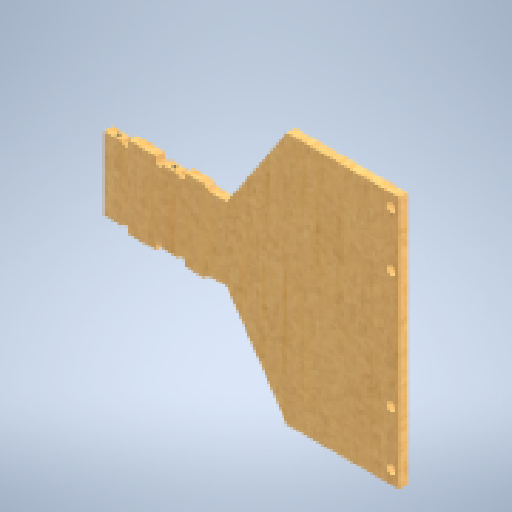
# Autodesk Inventor part: hera_porika2
Saved by Autodesk Inventor 2024 (Build 280153000, 153)
## iProperties
Created: 2024-01-03
Part Number: hera_porika2
Material: ポリカーボネート、クリア
Document SubType Name: Modeling
Designer: right
Density: 1.2 g/cm^3
Appearance: イエロー パイン材 - 硬質 塗装 抑えた光沢
Mass: 11.4076 g
Surface Area: 146.016 cm^2
Volume: 9.50636 cm^3
Author: right
Autodesk Inventor part; units mm, degrees
ref_plane "YZ Plane" through (0, 0, 0) normal (1, 0, 0) x (0, 1, 0)
ref_plane "XZ Plane" through (0, 0, 0) normal (0, 1, 0) x (-1, 0, 0)
ref_plane "XY Plane" through (0, 0, 0) normal (0, 0, 1) x (1, 0, 0)
sketch "スケッチ1" plane through (0, 0, 0) normal (0, 0, 1) x (1, 0, 0)
  line L0 (-10.8, 27.5) -> (31.8, 27.5)
  line L1 (31.8, 27.5) -> (31.8, 1.5)
  line L2 (31.8, 1.5) -> (-10.8, 1.5)
  line L3 (-10.8, 1.5) -> (-10.8, 27.5)
  line L4 (-35.2, 27.5) -> (27.8, 27.5) projected
  line L5 (-35.2, 1.5) -> (27.8, 1.5) projected
  line L6 (-8.3, 29) -> (-6.1, 29) projected
  line L7 (31.8, 1.5) -> (27.8, 1.5) projected
  ellipse E0 centre (-172.2553, 12.25) end of major axis (-172.2553, 4.25) minor radius 7.9976 projected
  line L8 (94.2, 59.5) -> (94.2, -30.5)
  line L9 (31.8, 14.5) -> (94.2, 14.5) construction
  line L10 (94.2, 59.5) -> (54.2, 59.5)
  line L11 (31.8, 27.5) -> (32.8, 27.5)
  line L12 (32.8, 27.5) -> (54.2, 59.5)
  circle A0 centre (32.2657, 28.5) radius 1
  line L13 (94.2, -30.5) -> (54.2, -30.5)
  line L14 (31.8, 2.9953) -> (54.2, -30.5)
  line L15 (0, 0) -> (5.6, 0) projected
  line L16 (5.6, 0) -> (5.6, 1.5) projected
  line L17 (0, 1.5) -> (5.6, 1.5) projected
  line L18 (0, 0) -> (0, 1.5) projected
  line L19 (-2.2, 1.5) -> (0, 1.5) projected
  line L20 (-2.2, 0) -> (0, 0) projected
  line L21 (5.6, 0) -> (7.8, 0) projected
  line L22 (11.7, 0) -> (13.9, 0) projected
  line L23 (17.8, 0) -> (20, 0) projected
  line L24 (20, 0) -> (25.6, 0) projected
  line L25 (25.6, 0) -> (27.8, 0) projected
  line L26 (17.8, 0) -> (17.8, 1.5)
  line L27 (31.8, 1.5) -> (32.8, 1.5)
  line L28 (27.8, 0) -> (27.8, 1.5)
  arc A1 (24.6775, 0) -> (27.8, 1.5) centre (24.6775, 4) ccw
  arc A2 (27.8, 1.5) -> (24.6775, 0) centre (27.8, -2.5) ccw
  circle A3 centre (16.7, 1.5) radius 1.1
  line L29 (7.8, 0) -> (7.8, 1.5)
  line L30 (-2.2, 0) -> (-2.2, 1.5)
  circle A4 centre (8.9, 1.5) radius 1.1
  circle A5 centre (-3.3, 1.5) radius 1.1
  line L31 (0, 29) -> (5.6, 29)
  line L32 (5.6, 29) -> (5.6, 27.5)
  line L33 (0, 29) -> (0, 27.5)
  line L34 (-2.2, 29) -> (0, 29)
  line L35 (11.7, 29) -> (13.9, 29)
  line L36 (17.8, 29) -> (20, 29)
  line L37 (20, 29) -> (25.6, 29)
  line L38 (25.6, 29) -> (27.8, 29)
  line L39 (17.8, 29) -> (17.8, 27.5)
  line L40 (27.8, 29) -> (27.8, 27.5)
  arc A6 (27.8, 27.5) -> (24.6775, 29) centre (24.6775, 25) ccw
  arc A7 (24.6775, 29) -> (27.8, 27.5) centre (27.8, 31.5) ccw
  circle A8 centre (16.7, 27.5) radius 1.1
  line L41 (-2.2, 29) -> (-2.2, 27.5)
  circle A9 centre (8.9, 27.5) radius 1.1
  line L42 (0, 29) -> (5.6, 29)
  line L43 (5.6, 29) -> (5.6, 27.5)
  line L44 (0, 29) -> (0, 27.5)
  line L45 (-2.2, 29) -> (0, 29)
  line L46 (5.6, 29) -> (7.8, 29)
  line L47 (7.8, 29) -> (7.8, 27.5)
  line L48 (-2.2, 29) -> (-2.2, 27.5)
  circle A10 centre (-3.3, 27.5) radius 1.1
  point P0 (15.6, 27.5)
  point P1 (10, 27.5)
  point P2 (7.8, 27.5)
  point P3 (-4.4, 1.5)
  point P4 (10, 1.5)
  point P5 (15.6, 1.5)
  point P6 (7.8, 27.5)
  point P7 (-4.4, 27.5)
  dimension "d7" = 2.2
  dimension "d8" = 2.2
  dimension "d9" = 2.2
  dimension "d0" = 2.5
  dimension "d2" = 1
  dimension "d3" = 2
  dimension "d4" = 90
  dimension "d5" = 40
  dimension "d6" = 4
  dimension "d39" = 105
  constraints: 68 end point, 24 symmetric about line, 12 point on line, 8 point on circle, 7 centre point, 5 horizontal, 4 perpendicular, 4 tangent, 3 parallel, 2 midpoint, 2 vertical, 17 other
  measures "d0" distance from line of L3 L6.start
  measures "d2" distance of L0.end L11.end
  measures "d3" diameter of A0
  measures "d4" distance of L8.start L8.end
  measures "d5" distance of L8.start L10.end
  measures "d6" radius of A1
  measures "d39" distance between parallel lines of L8 L3
extrude "押し出し1" add sketch "スケッチ1" along normal blind 3 contours L41 L34 L33 L0 | L0 A9 A8 L1 L2 A3 A4 A5 L3 A10 | L33 L31 L32 L0 | L32 L46 L47 L0 | L2 L18 L20 L30 | L39 L36 L37 A7 L0 | L2 L16 L15 L18 | L2 L29 L21 L16 | L11 L12 L10 L8 L13 L14 L1 | L14 L27 L1 | A2 L24 L23 L26 L2
fillet "フィレット1" radius 2 2 edges at (32.8, 27.5, 1.5) (32.8, 1.5, 1.5)
sketch "スケッチ2" plane through (0, 0, 0) normal (0, 0, -1) x (-1, 0, 0)
  arc A0 (-33.394, 28.3882) -> (-31.7315, 27.5) centre (-31.7315, 29.5) ccw projected
  arc A1 (-31.7315, 1.5) -> (-33.394, 0.6118) centre (-31.7315, -0.5) ccw projected
  line L0 (-33.394, 28.3882) -> (-33.394, 0.6118)
  line L1 (-54.2, 59.5) -> (-33.394, 28.3882) projected
  line L2 (-94.2, 59.5) -> (-54.2, 59.5) projected
  line L3 (-94.2, -30.5) -> (-94.2, 59.5) projected
  line L4 (-54.2, -30.5) -> (-94.2, -30.5) projected
  line L5 (-33.394, 0.6118) -> (-54.2, -30.5) projected
  arc A2 (-35.8877, 26.7205) -> (-34.1212, 25.1081) centre (-31.7315, 29.5) ccw
  line L6 (-35.8877, 26.7205) -> (-55.8028, 56.5)
  line L7 (-55.8028, 56.5) -> (-91.2, 56.5)
  line L8 (-91.2, 56.5) -> (-91.2, -27.5)
  line L9 (-91.2, -27.5) -> (-55.8028, -27.5)
  line L10 (-55.8028, -27.5) -> (-35.8877, 2.2795)
  arc A3 (-31.7315, 4.5) -> (-35.8877, 2.2795) centre (-31.7315, -0.5) ccw
  line L11 (-38.394, 30.4682) -> (-38.394, -1.4682)
  line L12 (-33.394, 24.4) -> (8.8, 24.4)
  line L13 (8.8, 24.4) -> (8.8, 4.6)
  line L14 (8.8, 4.6) -> (-33.394, 4.6)
  line L15 (-33.394, 4.6) -> (-33.394, 24.4)
  line L16 (10.8, 27.5) -> (10.8, 1.5) projected
  line L17 (-91.2, 14.5) -> (-38.394, 14.5) construction
  line L18 (-33.394, 24.4) -> (8.8, 4.6) construction
  line L19 (8.8, 24.4) -> (-33.394, 4.6) construction
  line L20 (-91.2, 14.5) -> (-45.8453, 41.6103) construction
  line L21 (-91.2, 14.5) -> (-45.8453, -12.6103) construction
  line L22 (-93.0741, 11.6323) -> (-42.432, 41.903)
  line L23 (-42.432, 41.903) -> (-43.9712, 44.478)
  line L24 (-43.9712, 44.478) -> (-94.6133, 14.2073)
  line L25 (-94.6133, 14.2073) -> (-93.0741, 11.6323)
  line L26 (-93.0741, 11.6323) -> (-43.9712, 44.478) construction
  line L27 (-42.432, 41.903) -> (-94.6133, 14.2073) construction
  line L28 (-90.9974, 16.1264) -> (-45.0103, -11.3618)
  line L29 (-46.6802, -13.8587) -> (-94.6133, 14.7927)
  line L30 (-33.395, 3.495) -> (9.6535, 23.696)
  line L31 (9.6535, 23.696) -> (8.8039, 25.5065)
  line L32 (8.8039, 25.5065) -> (-34.2446, 5.3055)
  line L33 (-34.2446, 5.3055) -> (-33.395, 3.495)
  line L34 (-33.395, 3.495) -> (8.8039, 25.5065) construction
  line L35 (9.6535, 23.696) -> (-34.2446, 5.3055) construction
  arc A4 (-15.6, 1.5) -> (-17.8, 1.5) centre (-16.7, 1.5) ccw projected
  arc A5 (-17.8, 27.5) -> (-15.6, 27.5) centre (-16.7, 27.5) ccw projected
  line L36 (8.3403, 3.7125) -> (-33.781, 23.4784)
  line L37 (-33.781, 23.4784) -> (-32.9314, 25.289)
  line L38 (-32.9314, 25.289) -> (9.1899, 5.5231)
  line L39 (9.1899, 5.5231) -> (8.3403, 3.7125)
  line L40 (8.3403, 3.7125) -> (-32.9314, 25.289) construction
  line L41 (-33.781, 23.4784) -> (9.1899, 5.5231) construction
  circle A6 centre (-91.2, 35.5) radius 3
  circle A7 centre (-91.2, 35.5) radius 1.6
  line L42 (-91.2, 56.5) -> (-91.2, 14.5) construction
  circle A8 centre (-91.2, 54.9) radius 3
  circle A9 centre (-91.2, 54.9) radius 1.6
  circle A10 centre (-91.2, -6.5) radius 3
  circle A11 centre (-91.2, -6.5) radius 1.6
  circle A12 centre (-91.2, -25.9) radius 3
  circle A13 centre (-91.2, -25.9) radius 1.6
  circle A14 centre (-73.2, -25.9) radius 1.6
  circle A15 centre (-73.2, -25.9) radius 3
  circle A16 centre (-73.2, 54.9) radius 3
  circle A17 centre (-73.2, 54.9) radius 1.6
  circle A18 centre (-55.2, -25.9) radius 1.6
  circle A19 centre (-55.2, -25.9) radius 3
  circle A20 centre (-55.2, 54.9) radius 3
  circle A21 centre (-55.2, 54.9) radius 1.6
  point P0 (0, 0)
  point P1 (-68.5226, 28.0551)
  point P2 (-93.0741, 17.3677)
  point P3 (-42.432, -12.903)
  point P4 (-43.9712, -15.478)
  point P5 (-12.297, 14.5)
  point P6 (-12.2956, 14.5007)
  point P7 (6.4459, 24.4)
  point P8 (8.8, 23.2954)
  point P9 (-31.0402, 4.6)
  point P10 (-33.394, 5.7047)
  point P11 (-42.7408, -13.697)
  point P12 (-91.2, 12.7525)
  point P13 (-88.2764, 14.5)
  point P14 (-41.3721, -10.9953)
  point P15 (-35.394, 1.2189)
  point P16 (-35.394, 27.7811)
  point P17 (-45.0103, 40.3618)
  point P18 (-91.2, 16.2475)
  point P19 (-46.6802, 42.8587)
  point P20 (-16.7, 2.6)
  point P21 (-16.7, 26.4)
  point P22 (-33.394, 5.7047)
  point P23 (-33.394, 3.4954)
  point P24 (6.4491, 4.6)
  point P25 (-12.2956, 13.3961)
  point P26 (-14.6495, 14.5007)
  point P27 (-33.394, 23.2968)
  point P28 (-9.9416, 14.5007)
  point P29 (8.8, 5.706)
  point P30 (-31.037, 24.4)
  point P31 (-12.2956, 15.6054)
  point P32 (-90.2, 15.4462)
  point P33 (-91.2, 12.7525)
  point P34 (-91.2, 35.5)
  point P35 (-91.2, -6.5)
  point P36 (-91.2, 33.9)
  point P37 (-91.2, 37.1)
  point P38 (-88.6623, 56.5)
  point P39 (-91.2, 51.9)
  point P40 (-91.2, 38.5)
  point P41 (-91.2, 32.5)
  point P42 (-91.2, 53.3)
  point P43 (-91.2, -9.5)
  point P44 (-91.2, -22.9)
  point P45 (-88.6623, -27.5)
  point P46 (-91.2, -3.5)
  point P47 (-91.2, -8.1)
  point P48 (-91.2, -4.9)
  point P49 (-57.7377, -27.5)
  point P50 (-53.2235, -23.6431)
  point P51 (-75.7377, -27.5)
  point P52 (-70.6623, -27.5)
  point P53 (-53.2235, 52.6431)
  point P54 (-57.7377, 56.5)
  point P55 (-70.6623, 56.5)
  point P56 (-75.7377, 56.5)
  point P57 (-55.74, 56.4061)
  point P58 (-54.0143, 53.8257)
  point P59 (-73.2, 56.5)
  point P60 (-55.74, -27.4061)
  point P61 (-54.0143, -24.8257)
  point P62 (-73.2, -27.5)
  dimension "d13" = 3
  dimension "d14" = 5
  dimension "d15" = 2
  dimension "d16" = 3
  dimension "d18" = 2
  dimension "d36" = 2
  dimension "d37" = 2
  dimension "d38" = 2
  dimension "d40" = 6
  dimension "d41" = 3.2
  dimension "d42" = 6
  dimension "d43" = 3.2
  dimension "d48" = 18
  constraints: 74 end point, 18 centre point, 13 midpoint, 12 parallel, 10 point on line, 9 coincident, 9 symmetric about line, 6 point on circle, 4 perpendicular, 3 horizontal, 3 tangent, 1 collinear, 1 vertical, 26 other
  measures "d13" distance between parallel lines of L1 L6
  measures "d14" distance between parallel lines of L0 L11
  measures "d15" distance between parallel lines of L16 L13
  measures "d16" distance of L23.end L22.end
  measures "d18" distance of L31.end L30.end
  measures "d36" distance from line of point (-16.7, 2.6) L14
  measures "d37" distance from line of L12 point (-16.7, 26.4)
  measures "d38" distance of L36.end L37.end
  measures "d40" diameter of A6
  measures "d41" diameter of A7
  measures "d42" diameter of A8
  measures "d43" diameter of A9
  measures "d48" distance of A13.centre A14.centre
extrude "押し出し2" cut sketch "スケッチ2" against normal blind 2 contours L6 L11 L10 L28 L22 | L36 L32 L0 | L12 L32 L38 | L24 L8 A6 A8 L7 A16 A20 L6 | A20 L7 L6 A21 | L29 L10 A19 L9 A15 A12 L8 A10 | L36 L14 L30 | L30 L13 L38 | A21 L6 | A17 | A16 L7 | L8 A7 | A11 L8 | L10 A18 L9 A19 | A9 L8 | L10 A18 | A14 | L9 A15 picked at (-57.4616, 56.0082) picked at (-55.2681, 54.3725) picked at (-70.697, 54.6556) picked at (-90.9686, 35.9805) picked at (-90.783, -6.1675) picked at (-57.4616, -27.0082) picked at (-90.7488, 55.3036) picked at (-55.4528, -26.2997) picked at (-70.697, -25.6556)
fillet "フィレット2" radius 2 29 edges at (91.2, 12.7525, 1) (88.2764, 14.5, 1) (91.2, 16.2475, 1) (46.6802, 42.8587, 1) (45.0103, 40.3618, 1) (33.394, 5.7047, 1) (31.0402, 4.6, 1) (-8.8, 23.2954, 1) (-6.4459, 24.4, 1) (33.394, 23.2968, 1) (31.037, 24.4, 1) (14.6495, 14.5007, 1) (12.2956, 15.6054, 1) (9.9416, 14.5007, 1) (12.2956, 13.3961, 1) (45.0103, -11.3618, 1) (46.6802, -13.8587, 1) (38.394, -1.4682, 1) (38.394, 30.4682, 1) (91.2, -3.5, 1) (91.2, -9.5, 1) (91.2, -22.9, 1) (88.6623, -27.5, 1) (91.2, 38.5, 1) (91.2, 32.5, 1) (91.2, 51.9, 1) (88.6623, 56.5, 1) (55.8028, -27.5, 1) (55.8028, 56.5, 1)
sketch "スケッチ3" plane through (10, 27.5, 0) normal (0, 1, 0) x (1, 0, 0)
  circle A0 centre (2.8, -1.5) radius 1.1 projected
  circle A1 centre (-17.2, -1.5) radius 1.1 projected
  point P0 (-10, 0)
  constraints: 2 coincident
hole "穴1" at (12.8, 27.5, 1.5) at (-7.2, 27.5, 1.5) direction (0, -1, 0) diameter 1.567 depth 4.5 tip angle 118 thread size "M2x0.4" class "6H" standard "ISO Metric profile"
sketch "スケッチ4" plane through (10, 1.5, 0) normal (0, -1, 0) x (1, 0, 0)
  arc A0 (2.1968, 2) -> (3.4032, 2) centre (2.8, 1.5) ccw projected
  circle A1 centre (-17.2, 1.5) radius 1.1 projected
  point P0 (-10, 0)
  point P1 (2.8, 1.5)
  constraints: 2 coincident
hole "穴2" at (12.8, 1.5, 1.5) at (-7.2, 1.5, 1.5) direction (0, 1, 0) diameter 1.567 depth 4.5 tip angle 118 thread size "M2x0.4" class "6H" standard "ISO Metric profile"
extrude "押し出し3" cut sketch "スケッチ2" against normal through all contours A7 L8 | L8 A7 | A11 L8 | L8 A11 | A9 L8 | L8 A9 | A13 L8 | L8 A13
